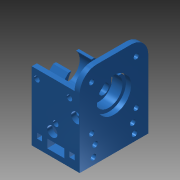
# Autodesk Inventor part: L bracket
Saved by Autodesk Inventor 2013 SP2 (Build 170200200, 200)
## iProperties
Created: 2017-05-18
Part Number: L bracket
Material: Generic
Document SubType Name: Modeling
Designer: Herman de Vries
Density: 1 g/cm^3
Author: Herman de Vries
Autodesk Inventor part; units mm, degrees
ref_plane "YZ Plane" through (0, 0, 0) normal (1, 0, 0) x (0, 1, 0)
ref_plane "XZ Plane" through (0, 0, 0) normal (0, 1, 0) x (-1, 0, 0)
ref_plane "XY Plane" through (0, 0, 0) normal (0, 0, 1) x (1, 0, 0)
sketch "Sketch1" plane through (0, 0, 0) normal (0, 0, 1) x (1, 0, 0)
  line L0 (0, 0) -> (28, 0)
  line L1 (28, 0) -> (28, 40)
  line L2 (28, 40) -> (0, 40)
  line L3 (0, 40) -> (0, 0)
  line L4 (9, 40) -> (19, 40)
  line L5 (19, 40) -> (19, 0)
  line L6 (19, 0) -> (9, 0)
  line L7 (9, 0) -> (9, 40)
  line L8 (9, 40) -> (6, 40)
  line L9 (6, 40) -> (6, 0)
  line L10 (6, 0) -> (9, 0)
  line L11 (9, 0) -> (9, 40)
  line L12 (19, 40) -> (22, 40)
  line L13 (22, 40) -> (22, 0)
  line L14 (22, 0) -> (19, 0)
  line L15 (19, 0) -> (19, 40)
  line L16 (25, 40) -> (28, 40)
  line L17 (28, 40) -> (28, 0)
  line L18 (28, 0) -> (25, 0)
  line L19 (25, 0) -> (25, 40)
  line L20 (9, 24) -> (19, 24)
  line L21 (19, 24) -> (19, 16)
  line L22 (19, 16) -> (9, 16)
  line L23 (9, 16) -> (9, 24)
  line L24 (9, 40) -> (19, 40)
  line L25 (19, 40) -> (19, 40)
  line L26 (19, 40) -> (9, 40)
  line L27 (9, 40) -> (9, 40)
  line L28 (9, 0) -> (19, 0)
  line L29 (19, 0) -> (19, 0)
  line L30 (19, 0) -> (9, 0)
  line L31 (9, 0) -> (9, 0)
  line L32 (0, 40) -> (3, 40)
  line L33 (3, 40) -> (3, 0)
  line L34 (3, 0) -> (0, 0)
  line L35 (0, 0) -> (0, 40)
  point P0 (14, 40)
  point P1 (14, 40)
  point P2 (9, 20)
  point P3 (9, 20)
  point P4 (9, 20)
  point P5 (0, 20)
  dimension "d0" = 28
  dimension "d1" = 40
  dimension "d15" = 10
  dimension "d16" = 40
  dimension "d18" = 3
  dimension "d19" = 3
  dimension "d20" = 3
  dimension "d30" = 8
  dimension "d33" = 3
  constraints: 72 end point, 18 equal length, 9 horizontal, 9 perpendicular, 7 collinear, 6 midpoint, 5 point on line, 2 coincident, 1 horizontal alignment
  measures "d0" distance of L2.end L1.end
  measures "d1" distance of L1.end L0.end
  measures "d15" distance of L4.start L4.end
  measures "d16" distance of L6.end L4.start
  measures "d18" distance of L9.end L10.end
  measures "d19" distance of L13.end L14.end
  measures "d20" distance of L17.end L18.end
  measures "d30" distance between parallel lines of L22 L20
  measures "d33" distance of L33.end L34.end
extrude "Extrusion1" add sketch "Sketch1" along normal blind 3
extrude "Extrusion3" add sketch "Sketch1" along normal blind 15 contours L3 L2 L33 L0 | L9 L2 L7 L0 | L5 L2 L13 L0
extrude "Extrusion4" add sketch "Sketch1" along normal blind 50 contours L19 L2 L1 L0
extrude "Extrusion6" add sketch "Sketch1" along normal blind 15 contours L7 L20 L5 L22
sketch "Sketch7" plane through (0, 0, 0) normal (-1, 0, 0) x (0, 0, 1)
  circle A0 centre (4, 32) radius 1.6
  circle A1 centre (4, 8) radius 1.6
  line L0 (4, 32) -> (4, 8) construction
  line L1 (15, 40) -> (15, 0) construction
  line L2 (0, 40) -> (15, 40) construction
  circle A2 centre (10, 31) radius 1.6
  circle A3 centre (10, 9) radius 1.6
  point P0 (0, 0)
  point P1 (4, 20)
  point P2 (15, 20)
  dimension "d34" = 3.2
  dimension "d35" = 3.2
  dimension "d36" = 24
  dimension "d40" = 4
  dimension "d48" = 3.2
  dimension "d49" = 3.2
  dimension "d50" = 9
  dimension "d51" = 5
  dimension "d52" = 5
  dimension "d53" = 9
  constraints: 4 centre point, 2 end point, 2 midpoint, 1 horizontal alignment, 1 vertical
  measures "d34" diameter of A0
  measures "d35" diameter of A1
  measures "d36" distance of L0.end L0.start
  measures "d40" horizontal distance of L2.start L0.start
  measures "d48" diameter of A2
  measures "d49" diameter of A3
  measures "d50" distance from line of A2.centre L2
  measures "d51" distance from line of A2.centre L1
  measures "d52" horizontal distance of A3.centre L1.end
  measures "d53" vertical distance of A3.centre L1.end
extrude "Extrusion7" cut sketch "Sketch7" against normal through all
sketch "Sketch9" plane through (0, 0, 3) normal (0, 0, 1) x (1, 0, 0)
  line L0 (3, 33.249) -> (6, 33.249) projected
  line L1 (6, 30.751) -> (3, 30.751) projected
  line L2 (6, 6.751) -> (3, 6.751) projected
  line L3 (3, 9.249) -> (6, 9.249) projected
  line L4 (3, 35) -> (6, 35)
  line L5 (6, 35) -> (6, 29)
  line L6 (6, 29) -> (3, 29)
  line L7 (3, 29) -> (3, 35)
  line L8 (22, 35) -> (25, 35)
  line L9 (25, 35) -> (25, 29)
  line L10 (25, 29) -> (22, 29)
  line L11 (22, 29) -> (22, 35)
  line L12 (3, 10.75) -> (6, 10.75)
  line L13 (6, 10.75) -> (6, 5.25)
  line L14 (6, 5.25) -> (3, 5.25)
  line L15 (3, 5.25) -> (3, 10.75)
  line L16 (22, 10.75) -> (25, 10.75)
  line L17 (25, 10.75) -> (25, 5.25)
  line L18 (25, 5.25) -> (22, 5.25)
  line L19 (22, 5.25) -> (22, 10.75)
  line L20 (3, 33.6) -> (3, 30.4) projected
  line L21 (3, 9.6) -> (3, 6.4) projected
  line L22 (22, 33.249) -> (25, 33.249) projected
  point P0 (0, 0)
  point P1 (4.5, 35)
  point P2 (4.5, 33.249)
  point P3 (23.5, 35)
  point P4 (3, 32)
  point P5 (3, 32)
  point P6 (3, 8)
  point P7 (3, 8)
  point P8 (23.5, 33.249)
  dimension "d41" = 6
  dimension "d43" = 5.5
  dimension "d44" = 3
  dimension "d45" = 3
  constraints: 32 end point, 8 collinear, 8 midpoint, 8 parallel, 4 horizontal, 4 perpendicular, 2 coincident, 2 vertical alignment
  measures "d41" distance of L6.end L4.start
  measures "d43" distance of L14.end L12.start
  measures "d44" distance of L12.start L12.end
  measures "d45" distance of L16.start L16.end
extrude "Extrusion8" cut sketch "Sketch9" against normal blind 5
sketch "Sketch10" plane through (0, 0, 0) normal (-1, 0, 0) x (0, 0, 1)
  circle A0 centre (10, 9) radius 1.6 construction
  circle A1 centre (10, 31) radius 1.6 construction
  circle A2 centre (10, 31) radius 3
  circle A3 centre (10, 9) radius 3
  dimension "d54" = 6
  dimension "d55" = 6
  constraints: 2 centre point, 2 coincident
  measures "d54" diameter of A2
  measures "d55" diameter of A3
extrude "Extrusion9" cut sketch "Sketch10" against normal blind 3
sketch "Sketch11" plane through (0, 0, 3) normal (0, 0, 1) x (1, 0, 0)
  line L0 (6, 5.25) -> (3, 5.25) projected
  line L1 (3, 5.25) -> (3, 0) projected
  line L2 (3, 0) -> (6, 0) projected
  line L3 (6, 0) -> (6, 5.25) projected
  line L4 (6, 29) -> (3, 29) projected
  line L5 (3, 29) -> (3, 10.75) projected
  line L6 (3, 10.75) -> (6, 10.75) projected
  line L7 (6, 10.75) -> (6, 29) projected
  line L8 (25, 5.25) -> (22, 5.25) projected
  line L9 (22, 5.25) -> (22, 0) projected
  line L10 (22, 0) -> (25, 0) projected
  line L11 (25, 0) -> (25, 5.25) projected
  line L12 (22, 10.75) -> (25, 10.75) projected
  line L13 (25, 10.75) -> (25, 29) projected
  line L14 (25, 29) -> (22, 29) projected
  line L15 (22, 29) -> (22, 10.75) projected
  line L16 (22, 35) -> (25, 35) projected
  line L17 (25, 35) -> (25, 40) projected
  line L18 (25, 40) -> (22, 40) projected
  line L19 (22, 40) -> (22, 35) projected
  line L20 (3, 35) -> (6, 35) projected
  line L21 (6, 35) -> (6, 40) projected
  line L22 (6, 40) -> (3, 40) projected
  line L23 (3, 40) -> (3, 35) projected
  point P0 (0, 0)
extrude "Extrusion10" add sketch "Sketch11" along normal blind 2
sketch "Sketch12" plane through (0, 0, 15) normal (0, 0, 1) x (1, 0, 0)
  line L0 (19, 40) -> (19, 24) construction
  line L1 (19, 24) -> (9, 24) construction
  line L2 (9, 24) -> (9, 40) construction
  line L3 (9, 40) -> (6, 40) construction
  line L4 (6, 40) -> (6, 0) construction
  line L5 (6, 0) -> (9, 0) construction
  line L6 (9, 0) -> (9, 16) construction
  line L7 (9, 16) -> (19, 16) construction
  line L8 (19, 16) -> (19, 0) construction
  line L9 (19, 0) -> (22, 0) construction
  line L10 (22, 0) -> (22, 40) construction
  line L11 (22, 40) -> (19, 40) construction
  line L12 (25, 40) -> (25, 0) construction
  line L13 (3, 0) -> (3, 40) construction
  line L14 (0, 40) -> (0, 0) construction
  line L15 (9, 37.5) -> (0, 37.5)
  line L16 (0, 37.5) -> (0, 2.5)
  line L17 (0, 2.5) -> (9, 2.5)
  line L18 (9, 2.5) -> (9, 37.5)
  line L19 (19, 37.5) -> (25, 37.5)
  line L20 (25, 37.5) -> (25, 2.5)
  line L21 (25, 2.5) -> (19, 2.5)
  line L22 (19, 2.5) -> (19, 37.5)
  point P0 (0, 20)
  point P1 (0, 20)
  point P2 (19, 20)
  point P3 (9, 20)
  dimension "d60" = 35
  constraints: 16 end point, 4 midpoint, 4 parallel, 4 point on line, 2 horizontal, 2 perpendicular, 1 coincident, 1 collinear, 1 horizontal alignment
  measures "d60" distance of L15.end L16.end
extrude "Extrusion11" add sketch "Sketch12" along normal blind 20
chamfer "Chamfer1" distance 10 angle 45 4 edges at (22, 37.5, 35) (4.5, 37.5, 35) (22, 2.5, 35) (4.5, 2.5, 35)
sketch "Sketch13" plane through (0, 0, 0) normal (-1, 0, 0) x (0, 0, 1)
  circle A0 centre (29.5, 20) radius 2.5 construction
  circle A1 centre (29.5, 20) radius 8
  dimension "d68" = 16
  constraints: 1 centre point, 1 coincident
  measures "d68" diameter of A1
extrude "Extrusion12" cut sketch "Sketch13" against normal blind 30
sketch "Sketch14" plane through (28, 0, 0) normal (1, 0, 0) x (0, 0, -1)
  circle A0 centre (-16.5, 7) radius 1.5 projected
  circle A1 centre (-42.5, 7) radius 1.5 projected
  circle A2 centre (-16.5, 33) radius 1.5 projected
  circle A3 centre (-42.5, 33) radius 1.5 projected
  circle A4 centre (-29.5, 20) radius 2.5 construction
  circle A5 centre (-29.5, 20) radius 10 projected
  point P0 (0, 0)
extrude "Extrusion13" cut sketch "Sketch14" against normal blind 3
fillet "Fillet1" radius 10 2 edges at (26.5, 40, 50) (26.5, 0, 50)
chamfer "Chamfer2" distance 2 angle 45 6 edges at (20.5, 40, 15) (7.5, 40, 15) (1.5, 40, 15) (7.5, 0, 15) (20.5, 0, 15) (1.5, 0, 15)
sketch "Sketch15" plane through (0, 0, 0) normal (0, -1, 0) x (1, 0, 0)
  line L0 (0, 8) -> (28, 8)
  line L1 (28, 8) -> (28, 40)
  line L2 (28, 40) -> (0, 40)
  line L3 (0, 40) -> (0, 8)
  line L4 (25, 40) -> (28, 40) projected
  line L5 (28, 0) -> (28, 40) projected
  line L6 (0, 0) -> (0, 13) projected
  dimension "d78" = 8
  constraints: 8 end point, 3 collinear, 2 parallel, 1 horizontal, 1 perpendicular
  measures "d78" distance from line of L6.start L0
extrude "Extrusion14" add sketch "Sketch15" against normal blind 3
sketch "Sketch16" plane through (0, 0, 0) normal (0, -1, 0) x (1, 0, 0)
  circle A0 centre (22, 35) radius 1.6
  circle A1 centre (3, 35) radius 1.6
  circle A2 centre (14, 18) radius 1.6
  line L0 (0, 0) -> (28, 0) projected
  circle A3 centre (12, 13) radius 1.6 construction
  circle A4 centre (26, 27) radius 1.6 construction
  circle A5 centre (12, 13) radius 3
  arc A6 (27.5, 29.5981) -> (27.5, 24.4019) centre (26, 27) ccw
  line L1 (28, 0) -> (28, 40) projected
  line L2 (3, 5) -> (3, 8) projected
  line L3 (27.5, 23.5581) -> (27.5, 30.9377)
  point P0 (14, 0)
  dimension "d81" = 3.2
  dimension "d82" = 3.2
  dimension "d83" = 3.2
  dimension "d84" = 35
  dimension "d85" = 3
  dimension "d86" = 6
  dimension "d87" = 18
  dimension "d104" = 6
  dimension "d105" = 6
  dimension "d107" = 0.5
  constraints: 5 centre point, 2 coincident, 2 end point, 2 point on circle, 2 point on line, 1 horizontal alignment, 1 midpoint, 1 parallel, 1 vertical alignment
  measures "d81" diameter of A0
  measures "d82" diameter of A1
  measures "d83" diameter of A2
  measures "d84" vertical distance of L0.start A1.centre
  measures "d85" horizontal distance of L0.start A1.centre
  measures "d86" horizontal distance of A0.centre L0.end
  measures "d87" distance from line of L0 A2.centre
  measures "d104" diameter of A5
  measures "d105" diameter of A6
  measures "d107" distance between parallel lines of L1 L3
extrude "Extrusion15" cut sketch "Sketch16" against normal blind 3
sketch "Sketch17" plane through (0, 0, 0) normal (-1, 0, 0) x (0, 0, 1)
  circle A0 centre (17, 21) radius 1.6 projected
  circle A1 centre (17, 21) radius 1.25
  circle A2 centre (17, 25) radius 1.25
  dimension "d91" = 2.5
  dimension "d94" = 2.5
  dimension "d96" = 4
  constraints: 2 centre point, 1 coincident, 1 vertical alignment
  measures "d91" diameter of A1
  measures "d94" diameter of A2
  measures "d96" distance of A2.centre A0.centre
extrude "Extrusion16" cut sketch "Sketch17" against normal blind 8 contours A1 | A2
sketch "Sketch18" plane through (0, 0, 15) normal (0, 0, -1) x (-1, 0, 0)
  line L0 (-6, 3) -> (-3, 3) projected
  line L1 (-3, 3) -> (-3, 37.5) projected
  line L2 (-6, 37.5) -> (-3, 37.5) projected
  line L3 (-6, 37.5) -> (-6, 3) projected
  line L4 (-25, 3) -> (-22, 3) projected
  line L5 (-22, 3) -> (-22, 37.5) projected
  line L6 (-22, 37.5) -> (-25, 37.5) projected
  line L7 (-25, 33) -> (-25, 37.5) projected
  line L8 (-25, 7) -> (-25, 33) projected
  line L9 (-25, 3) -> (-25, 7) projected
  point P0 (0, 0)
extrude "Extrusion17" cut sketch "Sketch18" against normal blind 5
sketch "Sketch19" plane through (0, 0, 0) normal (-1, 0, 0) x (0, 0, 1)
  circle A0 centre (16.5, 7) radius 1.5 projected
  circle A1 centre (16.5, 33) radius 1.5 projected
  circle A2 centre (16.5, 33) radius 3
  circle A3 centre (16.5, 7) radius 3
  point P0 (0, 0)
  dimension "d100" = 6
  dimension "d101" = 6
  constraints: 2 centre point, 2 coincident
  measures "d100" diameter of A2
  measures "d101" diameter of A3
extrude "Extrusion18" cut sketch "Sketch19" against normal up to surface (25 mm away) contours A0 | A1 | A2 | A3
equation "\"d34\" = d48"
equation "\"d35\" = d48"
equation "\"d49\" = d48"
equation "\"d52\" = d51"
equation "\"d53\" = d50"
equation "\"d81\" = d83"
equation "\"d82\" = d83"
body "Solid1"
